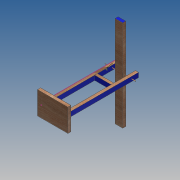
# Autodesk Inventor part: BrazoTFG
Saved by Autodesk Inventor 2014 (Build 180170000, 170)
## iProperties
Created: 2015-09-11
Part Number: BrazoTFG
Material: Madera (roble)
Document SubType Name: Modeling
Designer: yo
Density: 0.76 g/cm^3
Appearance: Abedul - Natural pulido
Author: yo
Autodesk Inventor part; units mm, degrees
ref_plane "YZ Plane" through (0, 0, 0) normal (1, 0, 0) x (0, 1, 0)
ref_plane "XZ Plane" through (0, 0, 0) normal (0, 1, 0) x (-1, 0, 0)
ref_plane "XY Plane" through (0, 0, 0) normal (0, 0, 1) x (1, 0, 0)
sketch "Boceto1" plane through (0, 0, 0) normal (0, 1, 0) x (-1, 0, 0)
  line L0 (-100, -75) -> (100, -75)
  line L1 (100, -75) -> (100, 75)
  line L2 (100, 75) -> (-100, 75)
  line L3 (-100, 75) -> (-100, -75)
  line L4 (-100, -75) -> (100, 75) construction
  line L5 (100, -75) -> (-100, 75) construction
  point P0 (0, 0)
  dimension "d0" = 200
  dimension "d1" = 150
  constraints: 12 end point, 2 midpoint, 2 parallel, 1 horizontal, 1 perpendicular
  measures "d0" distance of L2.end L1.end
  measures "d1" distance of L1.end L0.end
extrude "Extrusión1" add sketch "Boceto1" along normal blind 20
sketch "Boceto2" plane through (0, 20, 0) normal (0, 1, 0) x (1, 0, 0)
  line L0 (100, -75) -> (100, 75) projected
  line L1 (100, 0) -> (74, 0)
  line L2 (74, 0) -> (74, 15)
  line L3 (74, 15) -> (54, 15)
  line L4 (54, 15) -> (54, -15)
  line L5 (54, -15) -> (74, -15)
  line L6 (74, -15) -> (74, 0)
  line L7 (0, 0) -> (0, -60.8498)
  line L8 (-74, 0) -> (-74, 15)
  line L9 (-74, 15) -> (-54, 15)
  line L10 (-54, 15) -> (-54, -15)
  line L11 (-54, -15) -> (-74, -15)
  line L12 (-74, -15) -> (-74, 0)
  dimension "d4" = 26
  dimension "d5" = 15
  dimension "d6" = 20
  dimension "d7" = 30
  constraints: 24 end point, 5 symmetric about line, 3 parallel, 3 perpendicular, 1 collinear, 1 midpoint
  measures "d4" distance of L1.start L1.end
  measures "d5" distance of L1.end L2.end
  measures "d6" distance of L2.end L3.end
  measures "d7" distance of L3.end L4.end
extrude "Extrusión2" add sketch "Boceto2" along normal blind 470 separate body
sketch "Boceto3" plane through (54, 20, -15) normal (-1, 0, 0) x (0, 0, 1)
  line L0 (30, 0) -> (30, 470) projected
  line L1 (0, 0) -> (0, 470) projected
  line L2 (30, 470) -> (30, 328)
  line L3 (30, 328) -> (0, 328)
  line L4 (0, 328) -> (0, 310)
  line L5 (0, 310) -> (30, 310)
  point P0 (15, -20)
  dimension "d10" = 142
  dimension "d11" = 18
  constraints: 8 end point, 4 point on line, 2 perpendicular
  measures "d10" distance of L0.end L2.end
  measures "d11" distance of L3.end L4.end
extrude "Extrusión3" add sketch "Boceto3" along normal up to surface (108 mm away) separate body
sketch "Boceto4" plane through (-74, 20, -15) normal (-1, 0, 0) x (0, 0, 1)
  line L0 (0, 470) -> (30, 470) projected
  line L1 (0, 0) -> (0, 470) projected
  line L2 (15, 470) -> (15, 425)
  circle A0 centre (15, 425) radius 2
  point P0 (15, -20)
  dimension "d14" = 45
  dimension "d15" = 4
  constraints: 2 end point, 1 centre point, 1 coincident, 1 midpoint, 1 parallel
  measures "d14" distance of L2.start L2.end
  measures "d15" diameter of A0
sketch "Boceto5" plane through (-74, 20, -15) normal (-1, 0, 0) x (0, 0, 1)
  line L0 (0, 0) -> (30, 0) projected
  line L1 (30, 0) -> (30, 470) projected
  line L2 (0, 470) -> (30, 470) projected
  line L3 (0, 0) -> (0, 470) projected
  point P0 (15, -20)
hole "Hole1" at (-74, 445, 0) direction (1, 0, 0) diameter 4 end through all bodies 2
sketch "Boceto6" plane through (-74, 20, -15) normal (-1, 0, 0) x (0, 0, 1)
  circle A0 centre (15, 425) radius 2 projected
  line L0 (0, 0) -> (30, 0) projected
  line L1 (30, 0) -> (30, 470) projected
  line L2 (0, 470) -> (30, 470) projected
  line L3 (0, 0) -> (0, 470) projected
  circle A1 centre (15, 425) radius 2
  point P0 (15, -20)
  dimension "d23" = 4
  constraints: 1 centre point, 1 coincident
  measures "d23" diameter of A1
sketch "Boceto7" plane through (0, 0, 0) normal (1, 0, 0) x (0, 1, 0)
  circle A0 centre (445.0274, 0) radius 2
  point P0 (0, 0)
  dimension "d24" = 4
  constraints: 1 centre point
  measures "d24" diameter of A0
extrude "Extrusión4" add sketch "Boceto7" along normal blind 100 and the other way blind 100 separate body
sketch "Boceto8" plane through (0, 0, 0) normal (1, 0, 0) x (0, 1, 0)
  circle A0 centre (445.0274, 0) radius 2 projected
  line L0 (445.0274, 0) -> (455.0274, 0)
  line L1 (445.0274, 0) -> (445.0274, 300)
  line L2 (445.0274, 0) -> (445.0274, -300)
  line L3 (445.0274, -300) -> (455.0274, -300)
  line L4 (445.0274, -300) -> (435.0274, -300)
  line L5 (435.0274, -300) -> (435.0274, 300)
  line L6 (435.0274, 300) -> (455.0274, 300)
  line L7 (455.0274, 300) -> (455.0274, -300)
  point P0 (0, 0)
  dimension "d29" = 10
  dimension "d32" = 300
  dimension "d33" = 300
  dimension "d34" = 10
  dimension "d35" = 10
  dimension "d36" = 20
  constraints: 16 end point, 4 perpendicular, 2 collinear, 1 horizontal
  measures "d29" distance of L0.start L0.end
  measures "d32" distance of L0.start L1.end
  measures "d33" distance of L0.start L2.end
  measures "d34" distance of L2.end L3.end
  measures "d35" distance of L2.end L4.end
  measures "d36" distance of L5.end L6.end
extrude "Extrusión5" add sketch "Boceto8" along normal mid plane 50 separate body contours L0 L7 L3 L2 A0 | A0 L1 L6 L7 L0 | A0 L2 L4 L5 L6 L1
